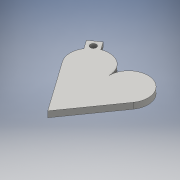
# Autodesk Inventor part: Gift - C
Saved by Autodesk Inventor 2016 (Build 200138000, 138)
## iProperties
Created: 2016-02-04
Part Number: Gift - C
Material: Generic
Document SubType Name: Modeling
Designer: TimB
Density: 1 g/cm^3
Appearance: Default
Author: TimB
Autodesk Inventor part; units mm, degrees
ref_plane "YZ Plane" through (0, 0, 0) normal (1, 0, 0) x (0, 1, 0)
ref_plane "XZ Plane" through (0, 0, 0) normal (0, 1, 0) x (-1, 0, 0)
ref_plane "XY Plane" through (0, 0, 0) normal (0, 0, 1) x (1, 0, 0)
sketch "Sketch1" plane through (0, 0, 0) normal (0, 0, 1) x (1, 0, 0)
  line L0 (0, -14) -> (-11.8124, 2.7546)
  line L1 (0, -14) -> (11.8124, 2.7546)
  arc A0 (0, 6.5) -> (-11.8124, 2.7546) centre (-6.5, 6.5) ccw
  arc A1 (11.8124, 2.7546) -> (0, 6.5) centre (6.5, 6.5) ccw
  point P0 (0, 0)
  constraints: 4 end point, 4 point on circle, 3 tangent, 2 centre point
extrude "Extrusion1" add sketch "Sketch1" along normal blind 2
sketch "Sketch4" plane through (0, 0, 2) normal (0, 0, 1) x (1, 0, 0)
  arc A0 (0, 6.5) -> (-11.8124, 2.7546) centre (-6.5, 6.5) ccw projected
  line L0 (-10.6694, 15.1841) -> (-13.9386, 12.8792)
  line L1 (-13.9386, 12.8792) -> (-11.9445, 10.0507)
  line L2 (-10.6694, 15.1841) -> (-8.8261, 12.5695)
  point P0 (0, 0)
  point P1 (0, -14)
  constraints: 6 end point, 2 point on circle, 1 parallel
extrude "Extrusion3" add sketch "Sketch4" against normal blind 1.5
sketch "Sketch5" plane through (0, 0, 0.5) normal (0, 0, -1) x (-1, 0, 0)
  line L0 (13.9386, 12.8792) -> (10.6694, 15.1841) projected
  arc A0 (11.8124, 2.7546) -> (0, 6.5) centre (6.5, 6.5) ccw projected
  circle A1 centre (11.1444, 12.3868) radius 1
  point P0 (0, 0)
  dimension "d14" = 2
  constraints: 1 centre point
  measures "d14" diameter of A1
hole "Hole1" at (-11.1444, 12.3868, 0.5) direction (0, 0, 1) diameter 2 end through all
sketch "Sketch6" plane through (0, 0, 0) normal (0, 0, -1) x (-1, 0, 0)
  line L0 (-11.8124, 2.7546) -> (0, -14) projected
  line L1 (11.8124, 2.7546) -> (0, -14) projected
  line L2 (0, -14) -> (0, -7)
  line L3 (-4.9352, -7) -> (4.9352, -7)
  spline S0 degree 2 poles (0.8335, -7.2139) (-1.6447, -7.2139) (-4.5506, -4.2188) (-4.5506, -1.5089) knots 0 0 0 1 2 2 2
  spline S1 degree 2 poles (-4.5506, -1.5089) (-4.5506, 1.1029) (-1.6357, 4.2139) (0.8424, 4.2139) knots 0 0 0 1 2 2 2
  spline S2 degree 2 poles (0.8424, 4.2139) (1.4931, 4.2139) (2.545, 4.0624) (3.0263, 3.9376) knots 0 0 0 1 2 2 2
  spline S3 degree 2 poles (3.0263, 3.9376) (3.4007, 3.8217) (4.2832, 3.4384) (4.5596, 3.2958) knots 0 0 0 1 2 2 2
  line L4 (4.5596, 3.2958) -> (4.5596, 0.675)
  line L5 (4.5596, 0.675) -> (4.2832, 0.675)
  spline S4 degree 2 poles (4.2832, 0.675) (4.0782, 0.8533) (3.472, 1.3525) (3.0887, 1.5843) knots 0 0 0 1 2 2 2
  spline S5 degree 2 poles (3.0887, 1.5843) (2.7054, 1.825) (1.7873, 2.1548) (1.2792, 2.1548) knots 0 0 0 1 2 2 2
  spline S6 degree 2 poles (1.2792, 2.1548) (0.6819, 2.1548) (-0.3075, 1.7804) (-0.7622, 1.3079) knots 0 0 0 1 2 2 2
  spline S7 degree 2 poles (-0.7622, 1.3079) (-1.1722, 0.889) (-1.6981, -0.5462) (-1.6981, -1.5178) knots 0 0 0 1 2 2 2
  spline S8 degree 2 poles (-1.6981, -1.5178) (-1.6981, -2.5429) (-1.1544, -3.9425) (-0.7087, -4.3703) knots 0 0 0 1 2 2 2
  spline S9 degree 2 poles (-0.7087, -4.3703) (-0.2808, -4.7893) (0.7711, -5.1548) (1.297, -5.1548) knots 0 0 0 1 2 2 2
  spline S10 degree 2 poles (1.297, -5.1548) (1.8408, -5.1548) (2.8302, -4.7893) (3.169, -4.5665) knots 0 0 0 1 2 2 2
  spline S11 degree 2 poles (3.169, -4.5665) (3.5434, -4.3436) (4.1049, -3.8712) (4.31, -3.684) knots 0 0 0 1 2 2 2
  line L6 (4.31, -3.684) -> (4.5596, -3.684)
  line L7 (4.5596, -3.684) -> (4.5596, -6.269)
  spline S12 degree 2 poles (4.5596, -6.269) (4.2565, -6.4117) (3.4631, -6.7682) (3.0353, -6.893) knots 0 0 0 1 2 2 2
  spline S13 degree 2 poles (3.0353, -6.893) (2.5182, -7.0535) (1.6179, -7.2139) (0.8335, -7.2139) knots 0 0 0 1 2 2 2
  point P0 (0, 0)
  dimension "d24" = 7
  constraints: 4 end point, 2 horizontal, 2 point on line, 1 vertical
  measures "d24" distance of L0.end L2.end
extrude "Extrusion5" add sketch "Sketch6" along normal blind 1 contours S0 S1 S2 S3 L4 L5 S4 S5 S6 S7 S8 S9 S10 S11 L6 L7 S12 S13 L3 | L3 L2 S0 | L2 L3 S13 S0
body "Solid1"
